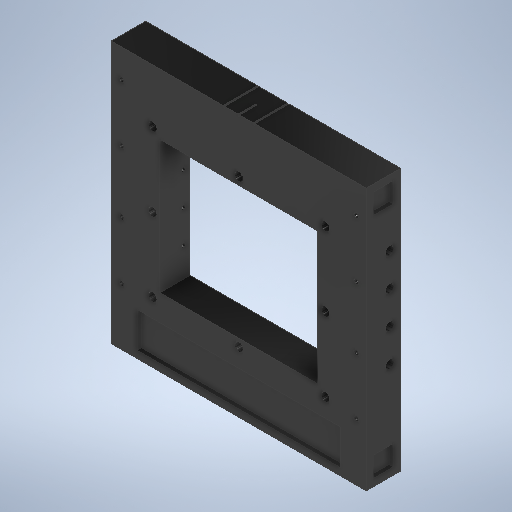
# Autodesk Inventor part: 22024_08_2110_Reaktorkorpus_hinten
Saved by Autodesk Inventor 2025.1 (Build 291241000, 241)
## iProperties
Created: 2020-09-23
Part Number: 22024_08_2110_Reaktorkorpus_hinten
Material: Acetalharz, Weiß
Document SubType Name: Modeling
Designer: Daniel
Density: 1.425 g/cm^3
Appearance: Glatt - Weiß
Author: Daniel
Autodesk Inventor part; units mm, degrees
(part 1 of 3)
ref_plane "YZ Plane" through (0, 0, 0) normal (1, 0, 0) x (0, 1, 0)
ref_plane "XZ Plane" through (0, 0, 0) normal (0, 1, 0) x (-1, 0, 0)
sketch "Skizze1" plane through (0, 0, 0) normal (0, 0, 1) x (1, 0, 0)
  line L0 (89, -91.5) -> (-89, -91.5)
  line L1 (-89, -91.5) -> (-89, 91.5)
  line L2 (-89, 91.5) -> (89, 91.5)
  line L3 (89, 91.5) -> (89, -91.5)
  line L4 (89, -91.5) -> (-89, 91.5) construction
  line L5 (-89, -91.5) -> (89, 91.5) construction
  point P0 (0, 0)
  dimension "d0" = 183
  dimension "d1" = 178
  constraints: 12 end point, 2 midpoint, 2 parallel, 1 horizontal, 1 perpendicular
  measures "d0" distance of L0.end L1.end
  measures "d1" distance of L1.end L2.end
extrude "Extrusion1" add sketch "Skizze1" along normal blind 24
sketch "Skizze2" plane through (0, 0, 24) normal (0, 0, 1) x (1, 0, 0)
  line L0 (-89, 91.5) -> (-89, -91.5) projected
  line L1 (-89, -91.5) -> (89, -91.5) projected
  line L2 (-89, 91.5) -> (89, 91.5)
  line L3 (89, 91.5) -> (89, -91.5)
  line L4 (89, -91.5) -> (-89, -91.5)
  line L5 (-89, -91.5) -> (-89, 91.5)
  line L6 (87, -89.5) -> (-87, -89.5)
  line L7 (-87, -89.5) -> (-87, 89.5)
  line L8 (-87, 89.5) -> (87, 89.5)
  line L9 (87, 89.5) -> (87, -89.5)
  line L10 (87, -89.5) -> (-87, 89.5) construction
  line L11 (-87, -89.5) -> (87, 89.5) construction
  line L12 (-70, -89.5) -> (70, -89.5)
  line L13 (70, -89.5) -> (70, 89.5)
  line L14 (70, 89.5) -> (-70, 89.5)
  line L15 (-70, 89.5) -> (-70, -89.5)
  line L16 (-70, -89.5) -> (70, 89.5) construction
  line L17 (70, -89.5) -> (-70, 89.5) construction
  line L18 (-65, -89.5) -> (65, -89.5)
  line L19 (65, -89.5) -> (65, 89.5)
  line L20 (65, 89.5) -> (-65, 89.5)
  line L21 (-65, 89.5) -> (-65, -89.5)
  line L22 (-65, -89.5) -> (65, 89.5) construction
  line L23 (65, -89.5) -> (-65, 89.5) construction
  line L24 (-65, 89.5) -> (-65, 91.5)
  line L25 (89, 91.5) -> (-89, 91.5) projected
  line L26 (-65, -89.5) -> (-65, -91.5)
  line L27 (65, -89.5) -> (65, -91.5)
  line L28 (65, 89.5) -> (65, 91.5)
  line L29 (89, -91.5) -> (89, 91.5) projected
  line L30 (-89, -91.5) -> (89, -91.5)
  line L31 (89, -91.5) -> (89, -86.5)
  line L32 (89, -86.5) -> (-89, -86.5)
  line L33 (-89, -86.5) -> (-89, -91.5)
  point P0 (0, 0)
  point P1 (70, -89.5)
  point P2 (87, -86.5)
  point P3 (70, -86.5)
  point P4 (-70, -86.5)
  point P5 (-87, -86.5)
  dimension "d4" = 2
  dimension "d5" = 2
  dimension "d6" = 17
  dimension "d7" = 24
  dimension "d10" = 5
  constraints: 60 end point, 11 parallel, 9 point on line, 6 midpoint, 6 perpendicular, 5 horizontal
  measures "d4" distance between parallel lines of L2 L8
  measures "d5" distance between parallel lines of L0 L7
  measures "d6" distance between parallel lines of L9 L13
  measures "d7" distance between parallel lines of L19 L3
  measures "d10" distance between parallel lines of L1 L32
extrude "Extrusion2" add sketch "Skizze2" along normal blind 156.5 contours L2 L24 L8 L7 L32 L0 | L32 L7 L6 L26 L1 L0 | L32 L15 L6 L7 | L2 L3 L32 L9 L8 L28 | L21 L32 L15 L8 | L32 L21 L6 L15 | L8 L13 L32 L19 | L27 L6 L9 L32 L3 L1 | L32 L13 L6 L19 | L9 L6 L13 L32
sketch "Skizze3" plane through (-89, 91.5, 0) normal (0, 1, 0) x (1, 0, 0)
  line L0 (0, 0) -> (0, -180.5) projected
  line L1 (0, -180.5) -> (55, -235.5)
  line L2 (0, -180.5) -> (24, -180.5) projected
  line L3 (24, -180.5) -> (-22.6667, -227.1667)
  line L4 (154, -24) -> (154, -180.5) projected
  line L5 (154, -180.5) -> (202, -228.5)
  line L6 (178, 0) -> (178, -180.5) projected
  line L7 (178, -180.5) -> (113.5, -245)
  line L8 (178, -180.5) -> (154, -180.5) projected
  line L9 (2, -24) -> (2, -180.5) projected
  line L10 (2, -180.5) -> (13, -191.5)
  line L11 (19, -180.5) -> (9.5, -190)
  line L12 (159, -24) -> (159, -180.5) projected
  line L13 (159, -180.5) -> (169, -189.5)
  line L14 (176, -24) -> (176, -180.5) projected
  line L15 (176, -180.5) -> (165, -191.5)
  point P0 (89, 0)
  point P1 (167.9474, -188.5526)
  point P2 (166, -192.5)
  point P3 (10.5, -189)
  point P4 (12, -192.5)
  dimension "d11" = 45
  dimension "d12" = 45
  dimension "d13" = 45
  dimension "d14" = 45
  constraints: 16 end point, 5 point on line, 3 perpendicular
  measures "d11" angle of L3 L2
  measures "d12" angle of L1 L2
  measures "d13" angle of L5 L8
  measures "d14" angle of L8 L7
extrude "Extrusion3" add sketch "Skizze3" against normal up to surface (183 mm away) contours L2 L10 L11 L1 | L11 L10 L3 L1 | L11 L2 L3 L10 | L8 L13 L15 L5 | L15 L13 L7 L5 | L15 L8 L7 L13
sketch "Skizze4" plane through (-89, -91.5, 0) normal (0, -1, 0) x (1, 0, 0)
  line L0 (19, 180.5) -> (10.5, 189) projected
  line L1 (10.5, 189) -> (19, 180.5)
  line L2 (2, 24) -> (2, 180.5) projected
  line L3 (19, 180.5) -> (2, 180.5)
  line L4 (10.5, 189) -> (2, 180.5) projected
  line L5 (2, 180.5) -> (10.5, 189)
  line L6 (167.9474, 188.5526) -> (159, 180.5) projected
  line L7 (176, 180.5) -> (167.9474, 188.5526) projected
  line L8 (159, 180.5) -> (167.9474, 188.5526)
  line L9 (159, 180.5) -> (176, 180.5) projected
  line L10 (167.9474, 188.5526) -> (176, 180.5)
  line L11 (176, 180.5) -> (159, 180.5)
  point P0 (89, 0)
  constraints: 12 end point, 2 collinear, 1 horizontal, 1 perpendicular
extrude "Extrusion4" add sketch "Skizze4" against normal blind 5
sketch "Skizze5" plane through (-89, 91.5, 0) normal (0, 1, 0) x (1, 0, 0)
  line L0 (10.5, -189) -> (2, -180.5) projected
  line L1 (2, -180.5) -> (10.5, -189)
  line L2 (10.5, -189) -> (19, -180.5)
  line L3 (19, -180.5) -> (10.5, -189) projected
  line L4 (2, -180.5) -> (19, -180.5)
  line L5 (167.9474, -188.5526) -> (159, -180.5) projected
  line L6 (176, -180.5) -> (167.9474, -188.5526) projected
  line L7 (159, -180.5) -> (176, -180.5)
  line L8 (159, -180.5) -> (167.9474, -188.5526)
  line L9 (176, -180.5) -> (167.9474, -188.5526)
  point P0 (89, 0)
  constraints: 13 end point, 3 collinear, 2 horizontal
extrude "Extrusion5" add sketch "Skizze5" against normal blind 2
sketch "Skizze6" plane through (0, 0, 0) normal (0, 0, -1) x (-1, 0, 0)
  line L0 (89, 91.5) -> (89, -91.5) projected
  line L1 (-89, -91.5) -> (89, -91.5)
  line L2 (89, -91.5) -> (89, -86.5)
  line L3 (89, -86.5) -> (-89, -86.5)
  line L4 (-89, -86.5) -> (-89, -91.5)
  line L5 (-89, -86.5) -> (89, -86.5)
  line L6 (89, -86.5) -> (89, -62.5)
  line L7 (89, -62.5) -> (-89, -62.5)
  line L8 (-89, -62.5) -> (-89, -86.5)
  line L9 (-89, -91.5) -> (-89, 91.5) projected
  line L10 (-89, 91.5) -> (89, 91.5)
  line L11 (89, 91.5) -> (89, 67.5)
  line L12 (89, 67.5) -> (-89, 67.5)
  line L13 (-89, 67.5) -> (-89, 91.5)
  line L14 (-89, 67.5) -> (89, -62.5) construction
  line L15 (89, 67.5) -> (-89, -62.5) construction
  line L16 (-75.35, -64) -> (75.35, -64)
  line L17 (75.35, -64) -> (75.35, 69)
  line L18 (75.35, 69) -> (-75.35, 69)
  line L19 (-75.35, 69) -> (-75.35, -64)
  line L20 (-75.35, -64) -> (75.35, 69) construction
  line L21 (75.35, -64) -> (-75.35, 69) construction
  point P0 (0, 0)
  point P1 (0, 2.5)
  dimension "d21" = 5
  dimension "d22" = 24
  dimension "d23" = 24
  dimension "d24" = 150.7
  dimension "d25" = 133
  constraints: 40 end point, 8 parallel, 4 horizontal, 4 perpendicular, 3 midpoint, 3 point on line
  measures "d21" distance between parallel lines of L1 L3
  measures "d22" distance between parallel lines of L3 L7
  measures "d23" distance between parallel lines of L12 L10
  measures "d24" distance of L17.end L18.end
  measures "d25" distance of L18.end L16.start
extrude "Extrusion6" cut sketch "Skizze6" against normal blind 3 contours L17 L7 L19 L12 | L12 L19 L18 L17 | L17 L16 L19 L7
sketch "Skizze7" plane through (0, 0, 3) normal (0, 0, -1) x (-1, 0, 0)
  line L0 (-75.35, 69) -> (75.35, -64) construction
  line L1 (75.35, -64) -> (75.35, 69) construction
  line L2 (75.35, 69) -> (-75.35, -64) construction
  line L3 (-55.1, 48.75) -> (55.1, 48.75)
  line L4 (55.1, 48.75) -> (55.1, -43.75)
  line L5 (55.1, -43.75) -> (-55.1, -43.75)
  line L6 (-55.1, -43.75) -> (-55.1, 48.75)
  line L7 (-55.1, 48.75) -> (55.1, -43.75) construction
  line L8 (55.1, 48.75) -> (-55.1, -43.75) construction
  line L9 (-75.35, 69) -> (75.35, 69) projected
  line L10 (75.35, -64) -> (-75.35, -64) projected
  line L11 (0, 2.5) -> (75.35, 2.5) construction
  line L12 (-75.35, -64) -> (-75.35, 69) projected
  line L13 (0, 2.5) -> (-75.35, 2.5) construction
  line L14 (-60.35, -49) -> (-60.35, 55.7618) construction
  line L15 (0, -49) -> (-60.35, -49) construction
  line L16 (0, -49) -> (60.35, -49) construction
  line L17 (60.35, -49) -> (60.35, 2.5) construction
  line L18 (60.35, 2.5) -> (60.35, 54) construction
  line L19 (60.35, 54) -> (0, 54) construction
  line L20 (0, 54) -> (60.35, 54) construction
  circle A0 centre (0, 54) radius 1.7
  circle A1 centre (60.35, 54) radius 1.7
  circle A2 centre (60.35, 2.5) radius 1.7
  circle A3 centre (60.35, -49) radius 1.7
  circle A4 centre (0, -49) radius 1.7
  circle A5 centre (-60.35, -49) radius 1.7
  circle A6 centre (-60.35, 2.5) radius 1.7
  line L21 (0, 54) -> (-60.35, 54) construction
  circle A7 centre (-60.35, 54) radius 1.7
  point P0 (-60.35, 2.5)
  point P1 (60.35, 2.5)
  point P2 (0, 0)
  dimension "d105" = 92.5
  dimension "d106" = 110.2
  dimension "d107" = 15
  dimension "d108" = 15
  dimension "d109" = 15
  dimension "d110" = 15
  dimension "d112" = 3.4
  dimension "d113" = 3.4
  dimension "d114" = 3.4
  dimension "d115" = 3.4
  dimension "d116" = 3.4
  dimension "d117" = 3.4
  dimension "d118" = 3.4
  dimension "d119" = 0
  dimension "d120" = 0
  dimension "d121" = 0
  dimension "d122" = 0
  dimension "d123" = 0
  dimension "d125" = 0
  dimension "d126" = 0
  dimension "d127" = 0
  dimension "d128" = 0
  dimension "d129" = 0
  dimension "d130" = 0
  dimension "d131" = 3.4
  dimension "d132" = 120.7
  dimension "d133" = 103
  dimension "d134" = 2.5
  constraints: 38 end point, 8 centre point, 7 point on line, 5 midpoint, 4 perpendicular, 2 horizontal, 2 parallel, 2 vertical
  measures "d105" distance of L5.end L3.start
  measures "d106" distance of L3.start L3.end
  measures "d107" distance from line of L9 L19.end
  measures "d108" distance from line of L10 L15.start
  measures "d109" distance from line of L17.end L1
  measures "d110" distance from line of L12 point (-60.35, 2.5)
  measures "d112" diameter of A0
  measures "d113" diameter of A1
  measures "d114" diameter of A2
  measures "d115" diameter of A3
  measures "d116" diameter of A4
  measures "d117" diameter of A5
  measures "d118" diameter of A6
  measures "d119" distance of L21.start L19.end
  measures "d120" distance of point (-60.35, 2.5) A6.centre
  measures "d121" distance of A4.centre L15.start
  measures "d122" distance of L17.end A2.centre
  measures "d123" distance from line of A6.centre L14
  measures "d125" distance of A5.centre L14.start
  measures "d126" distance of A5.centre L14.start
  measures "d127" distance of A3.centre L16.end
  measures "d128" distance of L16.end A3.centre
  measures "d129" distance of L18.end A1.centre
  measures "d130" distance of L18.end A1.centre
  measures "d131" diameter of A7
  measures "d132" distance of A2.centre A6.centre
  measures "d133" distance of A4.centre L21.start
  measures "d134" distance of point (0, 0) L11.start
extrude "Extrusion7" cut sketch "Skizze7" against normal through all
sketch "Skizze8" plane through (-89, -91.5, 0) normal (0, -1, 0) x (1, 0, 0)
  line L0 (0, 0) -> (0, 180.5) projected
  line L1 (24, 24) -> (24, 180.5) projected
  line L2 (0, 180.5) -> (24, 180.5)
  line L3 (24, 180.5) -> (24, 156.5)
  line L4 (24, 156.5) -> (0, 156.5)
  line L5 (0, 156.5) -> (0, 180.5)
  line L6 (154, 24) -> (154, 180.5) projected
  line L7 (178, 0) -> (178, 180.5) projected
  line L8 (154, 180.5) -> (178, 180.5)
  line L9 (178, 180.5) -> (178, 156.5)
  line L10 (178, 156.5) -> (154, 156.5)
  line L11 (154, 156.5) -> (154, 180.5)
  line L12 (178, 0) -> (0, 0) projected
  line L13 (178, 0) -> (154, 0)
  line L14 (154, 0) -> (154, 24)
  line L15 (154, 24) -> (178, 24)
  line L16 (178, 24) -> (178, 0)
  line L17 (0, 0) -> (24, 0)
  line L18 (24, 0) -> (24, 24)
  line L19 (24, 24) -> (0, 24)
  line L20 (0, 24) -> (0, 0)
  line L21 (0, 180.5) -> (24, 156.5) construction
  line L22 (24, 180.5) -> (0, 156.5) construction
  line L23 (154, 180.5) -> (178, 156.5) construction
  line L24 (178, 180.5) -> (154, 156.5) construction
  line L25 (154, 24) -> (178, 0) construction
  line L26 (178, 24) -> (154, 0) construction
  line L27 (0, 24) -> (24, 0) construction
  line L28 (24, 24) -> (0, 0) construction
  line L29 (5, 5) -> (19, 5)
  line L30 (19, 5) -> (19, 19)
  line L31 (19, 19) -> (5, 19)
  line L32 (5, 19) -> (5, 5)
  line L33 (5, 5) -> (19, 19) construction
  line L34 (19, 5) -> (5, 19) construction
  line L35 (159, 19) -> (173, 19)
  line L36 (173, 19) -> (173, 5)
  line L37 (173, 5) -> (159, 5)
  line L38 (159, 5) -> (159, 19)
  line L39 (159, 19) -> (173, 5) construction
  line L40 (173, 19) -> (159, 5) construction
  line L41 (159, 175.5) -> (173, 175.5)
  line L42 (173, 175.5) -> (173, 161.5)
  line L43 (173, 161.5) -> (159, 161.5)
  line L44 (159, 161.5) -> (159, 175.5)
  line L45 (159, 175.5) -> (173, 161.5) construction
  line L46 (173, 175.5) -> (159, 161.5) construction
  line L47 (5, 175.5) -> (19, 175.5)
  line L48 (19, 175.5) -> (19, 161.5)
  line L49 (19, 161.5) -> (5, 161.5)
  line L50 (5, 161.5) -> (5, 175.5)
  line L51 (5, 175.5) -> (19, 161.5) construction
  line L52 (19, 175.5) -> (5, 161.5) construction
  point P0 (89, 0)
  point P1 (12, 12)
  point P2 (166, 12)
  point P3 (166, 168.5)
  point P4 (12, 168.5)
  dimension "d38" = 24
  dimension "d39" = 24
  dimension "d40" = 14
  dimension "d41" = 14
  dimension "d187" = 14
  constraints: 96 end point, 16 parallel, 13 midpoint, 11 perpendicular, 10 point on line, 8 horizontal
  measures "d38" distance of L0.end L2.end
  measures "d39" distance between parallel lines of L4 L2
  measures "d40" distance of L47.start L47.end
  measures "d41" distance of L42.end L43.end
  measures "d187" distance of L35.start L35.end
extrude "Extrusion8" cut sketch "Skizze8" against normal blind 3 contours L32 L31 L30 L29 | L35 L36 L37 L38 | L41 L42 L43 L44 | L47 L48 L49 L50
ref_plane "Arbeitsebene1" through (77, 91.5, 192.5) normal (0, 0, -1) x (0, -1, 0)
sketch "Skizze9" plane through (77, 91.5, 192.5) normal (0, 0, -1) x (0, -1, 0)
  line L0 (183, -12) -> (0, -12) projected
  line L1 (183, 166) -> (178, 166)
  line L2 (178, 166) -> (178, -12)
  line L3 (178, -12) -> (183, -12)
  line L4 (183, -12) -> (183, 166)
  line L5 (183, 166) -> (183, -12) construction
  line L6 (183, 166) -> (178, -12) construction
  line L7 (183, -12) -> (178, 166) construction
  line L8 (180.5, 77) -> (134.2573, 77) construction
  line L9 (134.2573, 24.15) -> (134.2573, 129.85) construction
  line L10 (190.25, 79) -> (165.75, 79)
  line L11 (165.75, 79) -> (165.75, 75)
  line L12 (165.75, 75) -> (190.25, 75)
  line L13 (190.25, 75) -> (190.25, 79)
  line L14 (190.25, 79) -> (165.75, 75) construction
  line L15 (165.75, 79) -> (190.25, 75) construction
  line L16 (153.5, 148) -> (178, 148)
  line L17 (178, 148) -> (178, 6)
  line L18 (178, 6) -> (153.5, 6)
  line L19 (153.5, 6) -> (153.5, 148)
  line L20 (153.5, 148) -> (178, 6) construction
  line L21 (178, 148) -> (153.5, 6) construction
  line L22 (183, 142) -> (0, 142) projected
  line L23 (0, 12) -> (183, 12) projected
  point P0 (91.5, 77)
  point P1 (178, 77)
  point P2 (165.75, 77)
  point P3 (178, 148)
  dimension "d44" = 5
  dimension "d45" = 24.5
  dimension "d46" = 6
  dimension "d47" = 6
  constraints: 38 end point, 8 midpoint, 6 parallel, 3 horizontal, 3 perpendicular, 3 point on line
  measures "d44" distance between parallel lines of L4 L2
  measures "d45" distance of L11.end L12.end
  measures "d46" distance between parallel lines of L16 L22
  measures "d47" distance between parallel lines of L23 L18
extrude "Extrusion9" cut sketch "Skizze9" along normal up to surface (168.5 mm away) contours L18 L19 L23 L2 | L23 L19 L22 L2 L10 L11 L12 | L12 L11 L10 L2 | L19 L16 L2 L22
sketch "Skizze10" plane through (0, 0, 24) normal (0, 0, 1) x (1, 0, 0)
  line L0 (-71, -86.5) -> (-71, -62) construction
  line L1 (78.9474, -86.5) -> (71, -86.5) construction
  line L2 (-71, -62) -> (71, -86.5) construction
  line L3 (70, -62) -> (70, 89.5) construction
  line L4 (71, -86.5) -> (71, -61.9796) construction
  line L5 (71, -61.9796) -> (-71, -86.5) construction
  line L6 (-87, -86.5) -> (-65, -86.5) projected
  line L7 (-73.9133, -86.5) -> (-73.9133, -62)
  line L8 (-77, 91.5) -> (-77, -91.5) projected
  line L9 (-71, -62) -> (-65, -62) projected
  line L10 (-71, -62) -> (71, -62)
  line L11 (71, -62) -> (71, -86.5)
  line L12 (71, -86.5) -> (-71, -86.5)
  line L13 (-71, -86.5) -> (-71, -62)
  point P0 (0, 0)
  point P1 (0, -74.2398)
  constraints: 16 end point, 4 parallel, 1 horizontal, 1 midpoint, 1 perpendicular, 1 point on line
extrude "Extrusion10" cut sketch "Skizze10" against normal blind 3
sketch "Skizze11" plane through (-89, 91.5, 0) normal (0, 1, 0) x (1, 0, 0)
  line L0 (0, -180.5) -> (12, -192.5) projected
  line L1 (178, 0) -> (178, -180.5) projected
  line L2 (0, -180.5) -> (178, -180.5)
  line L3 (178, -180.5) -> (178, -178.5)
  line L4 (178, -178.5) -> (0, -178.5)
  line L5 (0, -178.5) -> (0, -180.5)
  line L6 (0, -180.5) -> (178, -178.5) construction
  line L7 (178, -180.5) -> (0, -178.5) construction
  line L8 (89, -179.5) -> (89, -173) construction
  line L9 (79, -190.75) -> (99, -190.75) construction
  line L10 (99, -190.75) -> (99, -166.25) construction
  line L11 (99, -166.25) -> (79, -166.25) construction
  line L12 (79, -166.25) -> (79, -190.75) construction
  line L13 (79, -190.75) -> (99, -166.25) construction
  line L14 (99, -190.75) -> (79, -166.25) construction
  line L15 (21, -154) -> (157, -154)
  line L16 (157, -154) -> (157, -178.5)
  line L17 (157, -178.5) -> (21, -178.5)
  line L18 (21, -178.5) -> (21, -154)
  line L19 (21, -154) -> (157, -178.5) construction
  line L20 (157, -154) -> (21, -178.5) construction
  line L21 (154, -24) -> (154, -180.5) projected
  line L22 (24, -24) -> (24, -180.5) projected
  point P0 (89, 0)
  point P1 (89, -178.5)
  point P2 (89, -166.25)
  point P3 (21, -178.5)
  dimension "d52" = 2
  dimension "d53" = 24.5
  dimension "d54" = 3
  dimension "d55" = 3
  constraints: 38 end point, 7 midpoint, 6 parallel, 3 horizontal, 3 perpendicular, 3 point on line, 1 vertical
  measures "d52" distance between parallel lines of L2 L4
  measures "d53" distance of L9.end L10.end
  measures "d54" distance between parallel lines of L16 L21
  measures "d55" distance between parallel lines of L18 L22
extrude "Extrusion11" cut sketch "Skizze11" against normal blind 181 contours L4 L21 L15 L16 | L4 L22 L15 L21 | L4 L18 L15 L22
sketch "Skizze12" plane through (77, 91.5, 192.5) normal (0, 0, -1) x (0, -1, 0)
  line L0 (178, 148) -> (153.5, 148) construction
  line L1 (153.5, 6) -> (178, 6) construction
  line L2 (153.5, 148) -> (178, 6) construction
  line L3 (178, 6) -> (153.5, 6) construction
  line L4 (153.5, 6) -> (178, 148) construction
  line L5 (165.75, 77) -> (145.75, 77) construction
  line L6 (145.75, 77) -> (145.75, 9) construction
  line L7 (0, 9) -> (153.5, 9) construction
  line L8 (145.75, 9) -> (145.75, 145) construction
  line L9 (0, 145) -> (153.5, 145) construction
  line L10 (135.75, 145) -> (135.75, 9) construction
  line L11 (135.75, 9) -> (125.75, 9) construction
  line L12 (125.75, 9) -> (125.75, 145) construction
  line L13 (115.75, 145) -> (115.75, 9) construction
  line L14 (115.75, 9) -> (105.75, 9) construction
  line L15 (105.75, 9) -> (105.75, 145) construction
  line L16 (95.75, 145) -> (95.75, 9) construction
  line L17 (95.75, 9) -> (85.75, 9) construction
  line L18 (85.75, 9) -> (85.75, 145) construction
  line L19 (75.75, 145) -> (75.75, 9) construction
  line L20 (75.75, 9) -> (65.75, 9) construction
  line L21 (65.75, 9) -> (65.75, 145) construction
  line L22 (55.75, 145) -> (55.75, 9) construction
  line L23 (45.75, 145) -> (45.75, 9) construction
  line L24 (35.75, 9) -> (35.75, 145) construction
  line L25 (25.75, 145) -> (25.75, 9) construction
  line L26 (15.75, 9) -> (15.75, 145) construction
  line L27 (149.75, 139) -> (141.75, 139)
  line L28 (141.75, 139) -> (141.75, 145)
  line L29 (141.75, 145) -> (149.75, 145)
  line L30 (149.75, 145) -> (149.75, 139)
  line L31 (149.75, 139) -> (141.75, 145) construction
  line L32 (141.75, 139) -> (149.75, 145) construction
  line L33 (141.75, 145) -> (143.75, 142)
  line L34 (149.75, 145) -> (147.75, 142)
  line L35 (153.5, 142) -> (0, 142) projected
  line L36 (143.75, 142) -> (147.75, 142)
  line L37 (0, 12) -> (153.5, 12) projected
  line L38 (149.75, 15) -> (141.75, 15)
  line L39 (141.75, 15) -> (141.75, 9)
  line L40 (141.75, 9) -> (149.75, 9)
  line L41 (149.75, 9) -> (149.75, 15)
  line L42 (149.75, 15) -> (141.75, 9) construction
  line L43 (141.75, 15) -> (149.75, 9) construction
  line L44 (149.75, 9) -> (147.75, 12)
  line L45 (141.75, 9) -> (143.75, 12)
  line L46 (143.75, 12) -> (147.75, 12)
  line L47 (131.75, 145) -> (139.75, 145)
  line L48 (131.75, 145) -> (133.75, 142)
  line L49 (139.75, 145) -> (137.75, 142)
  line L50 (133.75, 142) -> (137.75, 142)
  line L51 (131.75, 9) -> (139.75, 9)
  line L52 (139.75, 9) -> (137.75, 12)
  line L53 (131.75, 9) -> (133.75, 12)
  line L54 (133.75, 12) -> (137.75, 12)
  line L55 (121.75, 145) -> (129.75, 145)
  line L56 (121.75, 145) -> (123.75, 142)
  line L57 (129.75, 145) -> (127.75, 142)
  line L58 (123.75, 142) -> (127.75, 142)
  line L59 (121.75, 9) -> (129.75, 9)
  line L60 (129.75, 9) -> (127.75, 12)
  line L61 (121.75, 9) -> (123.75, 12)
  line L62 (123.75, 12) -> (127.75, 12)
  line L63 (111.75, 145) -> (119.75, 145)
  line L64 (111.75, 145) -> (113.75, 142)
  line L65 (119.75, 145) -> (117.75, 142)
  line L66 (113.75, 142) -> (117.75, 142)
  line L67 (111.75, 9) -> (119.75, 9)
  line L68 (119.75, 9) -> (117.75, 12)
  line L69 (111.75, 9) -> (113.75, 12)
  line L70 (113.75, 12) -> (117.75, 12)
  line L71 (101.75, 145) -> (109.75, 145)
  line L72 (101.75, 145) -> (103.75, 142)
  line L73 (109.75, 145) -> (107.75, 142)
  line L74 (103.75, 142) -> (107.75, 142)
  line L75 (101.75, 9) -> (109.75, 9)
  line L76 (109.75, 9) -> (107.75, 12)
  line L77 (101.75, 9) -> (103.75, 12)
  line L78 (103.75, 12) -> (107.75, 12)
  line L79 (91.75, 145) -> (99.75, 145)
  line L80 (91.75, 145) -> (93.75, 142)
  line L81 (99.75, 145) -> (97.75, 142)
  line L82 (93.75, 142) -> (97.75, 142)
  line L83 (91.75, 9) -> (99.75, 9)
  line L84 (99.75, 9) -> (97.75, 12)
  line L85 (91.75, 9) -> (93.75, 12)
  line L86 (93.75, 12) -> (97.75, 12)
  line L87 (81.75, 145) -> (89.75, 145)
  line L88 (81.75, 145) -> (83.75, 142)
  line L89 (89.75, 145) -> (87.75, 142)
  line L90 (83.75, 142) -> (87.75, 142)
  line L91 (81.75, 9) -> (89.75, 9)
  line L92 (89.75, 9) -> (87.75, 12)
  line L93 (81.75, 9) -> (83.75, 12)
  line L94 (83.75, 12) -> (87.75, 12)
  line L95 (71.75, 145) -> (79.75, 145)
  line L96 (71.75, 145) -> (73.75, 142)
  line L97 (79.75, 145) -> (77.75, 142)
  line L98 (73.75, 142) -> (77.75, 142)
  line L99 (71.75, 9) -> (79.75, 9)
  line L100 (79.75, 9) -> (77.75, 12)
  line L101 (71.75, 9) -> (73.75, 12)
  line L102 (73.75, 12) -> (77.75, 12)
  line L103 (61.75, 145) -> (69.75, 145)
  line L104 (61.75, 145) -> (63.75, 142)
  line L105 (69.75, 145) -> (67.75, 142)
  line L106 (63.75, 142) -> (67.75, 142)
  line L107 (61.75, 9) -> (69.75, 9)
  line L108 (69.75, 9) -> (67.75, 12)
  line L109 (61.75, 9) -> (63.75, 12)
  line L110 (63.75, 12) -> (67.75, 12)
  line L111 (51.75, 145) -> (59.75, 145)
  line L112 (51.75, 145) -> (53.75, 142)
  line L113 (59.75, 145) -> (57.75, 142)
  line L114 (53.75, 142) -> (57.75, 142)
  line L115 (51.75, 9) -> (59.75, 9)
  line L116 (59.75, 9) -> (57.75, 12)
  line L117 (51.75, 9) -> (53.75, 12)
  line L118 (53.75, 12) -> (57.75, 12)
  line L119 (41.75, 145) -> (49.75, 145)
  line L120 (41.75, 145) -> (43.75, 142)
  line L121 (49.75, 145) -> (47.75, 142)
  line L122 (43.75, 142) -> (47.75, 142)
  line L123 (41.75, 9) -> (49.75, 9)
  line L124 (49.75, 9) -> (47.75, 12)
  line L125 (41.75, 9) -> (43.75, 12)
  line L126 (43.75, 12) -> (47.75, 12)
  line L127 (31.75, 145) -> (39.75, 145)
  line L128 (31.75, 145) -> (33.75, 142)
  line L129 (39.75, 145) -> (37.75, 142)
  line L130 (33.75, 142) -> (37.75, 142)
  line L131 (31.75, 9) -> (39.75, 9)
  line L132 (39.75, 9) -> (37.75, 12)
  line L133 (31.75, 9) -> (33.75, 12)
  line L134 (33.75, 12) -> (37.75, 12)
  line L135 (21.75, 145) -> (29.75, 145)
  line L136 (21.75, 145) -> (23.75, 142)
  line L137 (29.75, 145) -> (27.75, 142)
  line L138 (23.75, 142) -> (27.75, 142)
  line L139 (21.75, 9) -> (29.75, 9)
  line L140 (29.75, 9) -> (27.75, 12)
  line L141 (21.75, 9) -> (23.75, 12)
  line L142 (23.75, 12) -> (27.75, 12)
  line L143 (11.75, 145) -> (19.75, 145)
  line L144 (11.75, 145) -> (13.75, 142)
  line L145 (19.75, 145) -> (17.75, 142)
  line L146 (13.75, 142) -> (17.75, 142)
  line L147 (11.75, 9) -> (19.75, 9)
  line L148 (19.75, 9) -> (17.75, 12)
  line L149 (11.75, 9) -> (13.75, 12)
  line L150 (13.75, 12) -> (17.75, 12)
  point P0 (91.5, 77)
  point P1 (145.75, 142)
  point P2 (145.75, 12)
  point P3 (135.75, 12)
  point P4 (125.75, 12)
  point P5 (115.75, 12)
  point P6 (105.75, 12)
  point P7 (95.75, 12)
  point P8 (85.75, 12)
  point P9 (75.75, 12)
  point P10 (65.75, 12)
  point P11 (55.75, 12)
  point P12 (45.75, 12)
  point P13 (35.75, 12)
  point P14 (25.75, 12)
  point P15 (15.75, 12)
  point P16 (135.75, 142)
  point P17 (125.75, 142)
  point P18 (115.75, 142)
  point P19 (105.75, 142)
  point P20 (95.75, 142)
  point P21 (85.75, 142)
  point P22 (75.75, 142)
  point P23 (65.75, 142)
  point P24 (55.75, 142)
  point P25 (45.75, 142)
  point P26 (35.75, 142)
  point P27 (25.75, 142)
  point P28 (15.75, 142)
  point P29 (125.75, 145)
  point P30 (115.75, 145)
  point P31 (105.75, 145)
  point P32 (95.75, 145)
  point P33 (85.75, 145)
  point P34 (75.75, 145)
  point P35 (65.75, 145)
  point P36 (35.75, 145)
  point P37 (25.75, 145)
  point P38 (15.75, 145)
  point P39 (13.75, 142)
  point P40 (17.75, 142)
  point P41 (23.75, 142)
  point P42 (27.75, 142)
  point P43 (33.75, 142)
  point P44 (37.75, 142)
  point P45 (17.75, 12)
  point P46 (13.75, 12)
  point P47 (27.75, 12)
  point P48 (23.75, 12)
  point P49 (37.75, 12)
  point P50 (33.75, 12)
  point P51 (43.75, 142)
  point P52 (47.75, 142)
  point P53 (53.75, 142)
  point P54 (57.75, 142)
  point P55 (63.75, 142)
  point P56 (67.75, 142)
  point P57 (73.75, 142)
  point P58 (77.75, 142)
  point P59 (83.75, 142)
  point P60 (107.75, 142)
  point P61 (43.75, 12)
  point P62 (57.75, 12)
  point P63 (53.75, 12)
  point P64 (63.75, 12)
  point P65 (87.75, 12)
  point P66 (97.75, 12)
  point P67 (93.75, 12)
  point P68 (107.75, 12)
  point P69 (103.75, 12)
  point P70 (113.75, 12)
  point P71 (127.75, 12)
  point P72 (123.75, 12)
  point P73 (117.75, 142)
  point P74 (123.75, 142)
  point P75 (127.75, 142)
  point P76 (133.75, 142)
  point P77 (137.75, 12)
  dimension "d58" = 20
  dimension "d59" = 10
  dimension "d60" = 10
  dimension "d61" = 10
  dimension "d62" = 10
  dimension "d63" = 10
  dimension "d64" = 10
  dimension "d65" = 10
  dimension "d66" = 10
  dimension "d67" = 10
  dimension "d68" = 10
  dimension "d69" = 10
  dimension "d70" = 10
  dimension "d71" = 10
  dimension "d72" = 8
  dimension "d73" = 2
  dimension "d74" = 2
  dimension "d75" = 8
  dimension "d76" = 2
  dimension "d77" = 2
  constraints: 290 end point, 36 point on line, 7 perpendicular, 5 midpoint, 5 parallel, 5 vertical, 4 horizontal, 1 collinear, 32 other
  measures "d58" distance of L5.start L5.end
  measures "d59" distance between parallel lines of L10 L8
  measures "d60" distance between parallel lines of L12 L10
  measures "d61" distance between parallel lines of L13 L12
  measures "d62" distance between parallel lines of L13 L15
  measures "d63" distance between parallel lines of L15 L16
  measures "d64" distance between parallel lines of L18 L16
  measures "d65" distance between parallel lines of L18 L19
  measures "d66" distance between parallel lines of L19 L21
  measures "d67" distance between parallel lines of L21 L22
  measures "d68" distance between parallel lines of L23 L22
  measures "d69" distance between parallel lines of L24 L23
  measures "d70" distance between parallel lines of L25 L24
  measures "d71" distance between parallel lines of L26 L25
  measures "d72" distance of L27.start L27.end
  measures "d73" distance from line of L28 L33.end
  measures "d74" distance from line of L30 L34.end
  measures "d75" distance of L38.start L38.end
  measures "d76" distance from line of L39 L45.end
  measures "d77" distance from line of L41 L44.end
extrude "Extrusion12" cut sketch "Skizze12" along normal blind 114 contours L35 L144 L143 L145 | L35 L136 L135 L137 | L35 L128 L127 L129 | L35 L120 L119 L121 | L35 L112 L111 L113 | L35 L104 L103 L105 | L35 L96 L95 L97 | L35 L88 L87 L89 | L35 L80 L79 L81 | L35 L72 L71 L73 | L35 L64 L63 L65 | L35 L56 L55 L57 | L35 L48 L47 L49 | L34 L35 L33 L29 | L37 L52 L51 L53 | L37 L60 L59 L61 | L37 L68 L67 L69 | L37 L76 L75 L77 | L37 L84 L83 L85 | L37 L92 L91 L93 | L37 L100 L99 L101 | L37 L108 L107 L109 | L37 L116 L115 L117 | L37 L124 L123 L125 | L37 L132 L131 L133 | L37 L140 L139 L141 | L37 L148 L147 L149 | L37 L44 L40 L45
sketch "Skizze13" plane through (-89, 91.5, 0) normal (0, 1, 0) x (1, 0, 0)
  line L0 (0, 0) -> (0, -180.5) projected
  line L1 (178, 0) -> (178, -180.5) projected
  line L2 (0, 0) -> (178, 0)
  line L3 (178, 0) -> (178, -178)
  line L4 (178, -178) -> (0, -178)
  line L5 (0, -178) -> (0, 0)
  line L6 (166, -192.5) -> (178, -180.5) projected
  line L7 (178, -178) -> (166, -178)
  line L8 (166, -178) -> (166, -192.5)
  line L9 (166, -192.5) -> (178, -192.5)
  line L10 (178, -192.5) -> (178, -178)
  line L11 (178, 0) -> (178, -180.5) construction
  line L12 (0, -178) -> (178, 0) construction
  line L13 (178, 0) -> (0, 0) construction
  line L14 (178, 0) -> (0, 0) construction
  line L15 (0, 0) -> (178, -178) construction
  line L16 (166, -89.5) -> (12, -89.5)
  line L17 (12, -89.5) -> (12, -88.5)
  line L18 (12, -88.5) -> (166, -88.5)
  line L19 (166, -88.5) -> (166, -89.5)
  line L20 (166, -89.5) -> (12, -88.5) construction
  line L21 (12, -89.5) -> (166, -88.5) construction
  line L22 (88.5, -166) -> (89.5, -166)
  line L23 (89.5, -166) -> (89.5, -12)
  line L24 (89.5, -12) -> (88.5, -12)
  line L25 (88.5, -12) -> (88.5, -166)
  line L26 (88.5, -166) -> (89.5, -12) construction
  line L27 (89.5, -166) -> (88.5, -12) construction
  line L28 (24, -154) -> (24, -24) projected
  line L29 (154, -154) -> (24, -154)
  line L30 (24, -154) -> (24, -24)
  line L31 (24, -24) -> (154, -24)
  line L32 (154, -24) -> (154, -154)
  line L33 (154, -154) -> (24, -24) construction
  line L34 (24, -154) -> (154, -24) construction
  point P0 (89, 0)
  point P1 (89, -89)
  point P2 (88.5, -88.5)
  point P3 (88.5, -89.5)
  point P4 (89.5, -89.5)
  point P5 (89.5, -88.5)
  dimension "d80" = 178
  dimension "d81" = 14.5
  dimension "d82" = 1
  dimension "d83" = 1
  dimension "d84" = 154
  dimension "d85" = 154
  dimension "d90" = 130
  dimension "d91" = 130
  constraints: 58 end point, 11 equal length, 7 midpoint, 5 horizontal, 5 perpendicular, 1 point on line
  measures "d80" distance between parallel lines of L4 L2
  measures "d81" distance between parallel lines of L4 L9
  measures "d82" distance of L16.end L17.end
  measures "d83" distance of L23.end L24.end
  measures "d84" distance of L24.end L22.start
  measures "d85" distance of L17.end L18.end
  measures "d90" distance of L28.end L31.end
  measures "d91" distance of L29.end L28.end
extrude "Extrusion13" cut sketch "Skizze13" against normal blind 1 contours L16 L32 L18 L19 | L16 L23 L18 L32 | L23 L29 L25 L16 | L16 L25 L18 L23 | L16 L28 L18 L25 | L23 L22 L25 L29 | L18 L25 L31 L23 | L16 L17 L18 L28 | L31 L25 L24 L23
sketch "Skizze14" plane through (-77, -91.5, 192.5) normal (0.7071, 0, 0.7071) x (0.7071, 0, -0.7071)
  line L0 (0.4493, 19.9089) -> (5.7022, 19.9089) construction
  line L1 (5.7022, 19.9089) -> (5.7022, 29.9599) construction
  line L2 (5.7022, 29.9599) -> (0.4493, 29.9599) construction
  line L3 (0.4493, 29.9599) -> (0.4493, 19.9089) construction
  line L4 (0.4923, 49.8867) -> (5.7451, 49.8867) construction
  line L5 (5.7451, 49.8867) -> (5.7451, 46.2392) construction
  line L6 (5.7451, 46.2392) -> (0.4923, 46.2392) construction
  line L7 (0.4923, 46.2392) -> (0.4923, 49.8867) construction
  line L8 (0.1277, 60.4817) -> (5.3805, 60.4817) construction
  line L9 (5.3805, 60.4817) -> (5.3805, 56.8342) construction
  line L10 (5.3805, 56.8342) -> (0.1277, 56.8342) construction
  line L11 (0.1277, 56.8342) -> (0.1277, 60.4817) construction
  line L12 (0.177, 70.1367) -> (5.4298, 70.1367) construction
  line L13 (5.4298, 70.1367) -> (5.4298, 66.4892) construction
  line L14 (5.4298, 66.4892) -> (0.177, 66.4892) construction
  line L15 (0.177, 66.4892) -> (0.177, 70.1367) construction
  line L16 (0.177, 80.1367) -> (5.4298, 80.1367) construction
  line L17 (5.4298, 80.1367) -> (5.4298, 76.4892) construction
  line L18 (5.4298, 76.4892) -> (0.177, 76.4892) construction
  line L19 (0.177, 76.4892) -> (0.177, 80.1367) construction
  line L20 (0.177, 90.1367) -> (5.4298, 90.1367) construction
  line L21 (5.4298, 90.1367) -> (5.4298, 86.4892) construction
  line L22 (5.4298, 86.4892) -> (0.177, 86.4892) construction
  line L23 (0.177, 86.4892) -> (0.177, 90.1367) construction
  line L24 (0.177, 100.1367) -> (5.4298, 100.1367) construction
  line L25 (5.4298, 100.1367) -> (5.4298, 96.4892) construction
  line L26 (5.4298, 96.4892) -> (0.177, 96.4892) construction
  line L27 (0.177, 96.4892) -> (0.177, 100.1367) construction
  line L28 (0.177, 110.1367) -> (5.4298, 110.1367) construction
  line L29 (5.4298, 110.1367) -> (5.4298, 106.4892) construction
  line L30 (5.4298, 106.4892) -> (0.177, 106.4892) construction
  line L31 (0.177, 106.4892) -> (0.177, 110.1367) construction
  line L32 (-0.2126, 120.6134) -> (5.0402, 120.6134) construction
  line L33 (5.0402, 120.6134) -> (5.0402, 116.9659) construction
  line L34 (5.0402, 116.9659) -> (-0.2126, 116.9659) construction
  line L35 (-0.2126, 116.9659) -> (-0.2126, 120.6134) construction
  line L36 (-0.2161, 130.1063) -> (5.0368, 130.1063) construction
  line L37 (5.0368, 130.1063) -> (5.0368, 126.4588) construction
  line L38 (5.0368, 126.4588) -> (-0.2161, 126.4588) construction
  line L39 (-0.2161, 126.4588) -> (-0.2161, 130.1063) construction
  line L40 (-0.2978, 140.1) -> (4.9551, 140.1) construction
  line L41 (4.9551, 140.1) -> (4.9551, 136.4525) construction
  line L42 (4.9551, 136.4525) -> (-0.2978, 136.4525) construction
  line L43 (-0.2978, 136.4525) -> (-0.2978, 140.1) construction
  line L44 (-0.3019, 150.1519) -> (4.9509, 150.1519) construction
  line L45 (4.9509, 150.1519) -> (4.9509, 146.5044) construction
  line L46 (4.9509, 146.5044) -> (-0.3019, 146.5044) construction
  line L47 (-0.3019, 146.5044) -> (-0.3019, 150.1519) construction
  line L48 (-0.2744, 160.1018) -> (4.9784, 160.1018) construction
  line L49 (4.9784, 160.1018) -> (4.9784, 156.4543) construction
  line L50 (4.9784, 156.4543) -> (-0.2744, 156.4543) construction
  line L51 (-0.2744, 156.4543) -> (-0.2744, 160.1018) construction
  line L52 (-0.539, 170.1317) -> (4.1973, 170.1317) construction
  line L53 (4.1973, 170.1317) -> (4.1973, 166.4842) construction
  line L54 (4.1973, 166.4842) -> (-0.539, 166.4842) construction
  line L55 (-0.539, 166.4842) -> (-0.539, 170.1317) construction
  line L56 (0.5265, 39.54) -> (5.7793, 39.54) construction
  line L57 (5.7793, 39.54) -> (5.7793, 35.8925) construction
  line L58 (5.7793, 35.8925) -> (0.5265, 35.8925) construction
  line L59 (0.5265, 35.8925) -> (0.5265, 39.54) construction
  line L60 (8.4853, 5) -> (8.4853, 29.5) projected
  line L61 (12.1672, 16.75) -> (4.8034, 16.75)
  line L62 (4.8034, 16.75) -> (4.8034, 17.75)
  line L63 (4.8034, 17.75) -> (12.1672, 17.75)
  line L64 (12.1672, 17.75) -> (12.1672, 16.75)
  line L65 (12.1672, 16.75) -> (4.8034, 17.75) construction
  line L66 (4.8034, 16.75) -> (12.1672, 17.75) construction
  line L67 (7.3114, 17.75) -> (7.3114, 16.75)
  line L68 (2.9776, 164.5202) -> (0.2945, 164.5202)
  line L69 (0.2945, 164.5202) -> (0.2945, 165.0818)
  line L70 (0.2945, 165.0818) -> (1.2928, 165.0818)
  line L71 (1.2928, 165.0818) -> (1.2928, 168.7678)
  line L72 (1.2928, 168.7678) -> (0.2945, 168.7678)
  line L73 (0.2945, 168.7678) -> (0.2945, 169.2715)
  spline S0 degree 2 poles (0.2945, 169.2715) (0.8605, 169.2715) (1.3954, 169.5924) (1.431, 170.0381) knots 0 0 0 1 2 2 2
  line L74 (1.431, 170.0381) -> (2.0015, 170.0381)
  line L75 (2.0015, 170.0381) -> (2.0015, 165.0818)
  line L76 (2.0015, 165.0818) -> (2.9776, 165.0818)
  line L77 (2.9776, 165.0818) -> (2.9776, 164.5202)
  spline S1 degree 2 poles (7.4659, 166.3031) (7.4659, 165.8796) (7.1851, 165.1621) (6.9488, 164.9214) knots 0 0 0 1 2 2 2
  spline S2 degree 2 poles (6.9488, 164.9214) (6.7037, 164.6673) (6.0886, 164.4044) (5.7187, 164.4044) knots 0 0 0 1 2 2 2
  spline S3 degree 2 poles (5.7187, 164.4044) (5.3488, 164.4044) (4.7381, 164.6539) (4.5064, 164.9035) knots 0 0 0 1 2 2 2
  spline S4 degree 2 poles (4.5064, 164.9035) (4.2211, 165.2022) (3.9002, 166.205) (3.9002, 166.936) knots 0 0 0 1 2 2 2
  spline S5 degree 2 poles (3.9002, 166.936) (3.9002, 167.6535) (4.1944, 168.8079) (4.5019, 169.2358) knots 0 0 0 1 2 2 2
  spline S6 degree 2 poles (4.5019, 169.2358) (4.8005, 169.6548) (5.7454, 170.1227) (6.365, 170.1227) knots 0 0 0 1 2 2 2
  spline S7 degree 2 poles (6.365, 170.1227) (6.5477, 170.1227) (6.8686, 170.0871) (6.989, 170.047) knots 0 0 0 1 2 2 2
  line L78 (6.989, 170.047) -> (6.989, 169.3383)
  line L79 (6.989, 169.3383) -> (6.9578, 169.3383)
  spline S8 degree 2 poles (6.9578, 169.3383) (6.8552, 169.3918) (6.4808, 169.4854) (6.2669, 169.4854) knots 0 0 0 1 2 2 2
  spline S9 degree 2 poles (6.2669, 169.4854) (5.5805, 169.4854) (4.7381, 168.5583) (4.6579, 167.6491) knots 0 0 0 1 2 2 2
  spline S10 degree 2 poles (4.6579, 167.6491) (4.9209, 167.8318) (5.4736, 168.0324) (5.8034, 168.0324) knots 0 0 0 1 2 2 2
  spline S11 degree 2 poles (5.8034, 168.0324) (6.1243, 168.0324) (6.6056, 167.9031) (6.8686, 167.707) knots 0 0 0 1 2 2 2
  spline S12 degree 2 poles (6.8686, 167.707) (7.1717, 167.4797) (7.4659, 166.7755) (7.4659, 166.3031) knots 0 0 0 1 2 2 2
  spline S13 degree 2 poles (6.7171, 166.2719) (6.7171, 166.6106) (6.5388, 167.0697) (6.3427, 167.2301) knots 0 0 0 1 2 2 2
  spline S14 degree 2 poles (6.3427, 167.2301) (6.1956, 167.346) (5.8301, 167.4218) (5.6385, 167.4218) knots 0 0 0 1 2 2 2
  spline S15 degree 2 poles (5.6385, 167.4218) (5.38, 167.4218) (4.8941, 167.2658) (4.6579, 167.1187) knots 0 0 0 1 2 2 2
  spline S16 degree 2 poles (4.6579, 167.1187) (4.6535, 167.0385) (4.6445, 166.8869) (4.6445, 166.771) knots 0 0 0 1 2 2 2
  spline S17 degree 2 poles (4.6445, 166.771) (4.6445, 166.2005) (4.8674, 165.5008) (5.0368, 165.318) knots 0 0 0 1 2 2 2
  spline S18 degree 2 poles (5.0368, 165.318) (5.1928, 165.1442) (5.5315, 165.0061) (5.7231, 165.0061) knots 0 0 0 1 2 2 2
  spline S19 degree 2 poles (5.7231, 165.0061) (6.1689, 165.0061) (6.7171, 165.639) (6.7171, 166.2719) knots 0 0 0 1 2 2 2
  spline S20 degree 2 poles (11.5396, 167.2702) (11.5396, 165.7905) (10.6794, 164.4044) (9.7835, 164.4044) knots 0 0 0 1 2 2 2
  spline S21 degree 2 poles (9.7835, 164.4044) (8.8743, 164.4044) (8.023, 165.8172) (8.023, 167.2658) knots 0 0 0 1 2 2 2
  spline S22 degree 2 poles (8.023, 167.2658) (8.023, 168.7544) (8.8832, 170.1317) (9.7835, 170.1317) knots 0 0 0 1 2 2 2
  spline S23 degree 2 poles (9.7835, 170.1317) (10.6883, 170.1317) (11.5396, 168.7054) (11.5396, 167.2702) knots 0 0 0 1 2 2 2
  spline S24 degree 2 poles (10.5947, 165.5944) (10.7017, 165.8663) (10.7908, 166.7042) (10.7908, 167.2702) knots 0 0 0 1 2 2 2
  spline S25 degree 2 poles (10.7908, 167.2702) (10.7908, 167.8363) (10.7017, 168.6697) (10.5902, 168.9505) knots 0 0 0 1 2 2 2
  spline S26 degree 2 poles (10.5902, 168.9505) (10.4788, 169.2313) (10.0911, 169.521) (9.7835, 169.521) knots 0 0 0 1 2 2 2
  spline S27 degree 2 poles (9.7835, 169.521) (9.476, 169.521) (9.0793, 169.2313) (8.9634, 168.9416) knots 0 0 0 1 2 2 2
  spline S28 degree 2 poles (8.9634, 168.9416) (8.852, 168.6608) (8.7718, 167.8051) (8.7718, 167.2658) knots 0 0 0 1 2 2 2
  spline S29 degree 2 poles (8.7718, 167.2658) (8.7718, 166.6864) (8.8431, 165.9108) (8.959, 165.6078) knots 0 0 0 1 2 2 2
  spline S30 degree 2 poles (8.959, 165.6078) (9.0659, 165.3225) (9.4626, 165.015) (9.7835, 165.015) knots 0 0 0 1 2 2 2
  spline S31 degree 2 poles (9.7835, 165.015) (10.0866, 165.015) (10.4833, 165.3047) (10.5947, 165.5944) knots 0 0 0 1 2 2 2
  line L80 (3.2422, 154.4903) -> (0.559, 154.4903)
  line L81 (0.559, 154.4903) -> (0.559, 155.0519)
  line L82 (0.559, 155.0519) -> (1.5574, 155.0519)
  line L83 (1.5574, 155.0519) -> (1.5574, 158.7379)
  line L84 (1.5574, 158.7379) -> (0.559, 158.7379)
  line L85 (0.559, 158.7379) -> (0.559, 159.2416)
  spline S32 degree 2 poles (0.559, 159.2416) (1.1251, 159.2416) (1.6599, 159.5625) (1.6956, 160.0082) knots 0 0 0 1 2 2 2
  line L86 (1.6956, 160.0082) -> (2.2661, 160.0082)
  line L87 (2.2661, 160.0082) -> (2.2661, 155.0519)
  line L88 (2.2661, 155.0519) -> (3.2422, 155.0519)
  line L89 (3.2422, 155.0519) -> (3.2422, 154.4903)
  spline S33 degree 2 poles (7.5878, 156.2375) (7.5878, 155.8408) (7.3337, 155.1634) (7.102, 154.9138) knots 0 0 0 1 2 2 2
  spline S34 degree 2 poles (7.102, 154.9138) (6.8702, 154.6642) (6.1794, 154.3745) (5.7515, 154.3745) knots 0 0 0 1 2 2 2
  spline S35 degree 2 poles (5.7515, 154.3745) (5.3593, 154.3745) (4.5927, 154.5483) (4.3119, 154.6865) knots 0 0 0 1 2 2 2
  line L90 (4.3119, 154.6865) -> (4.3119, 155.4664)
  line L91 (4.3119, 155.4664) -> (4.3653, 155.4664)
  spline S36 degree 2 poles (4.3653, 155.4664) (4.45, 155.404) (4.7665, 155.2436) (4.9581, 155.1723) knots 0 0 0 1 2 2 2
  spline S37 degree 2 poles (4.9581, 155.1723) (5.1765, 155.0965) (5.5375, 155.0118) (5.7649, 155.0118) knots 0 0 0 1 2 2 2
  spline S38 degree 2 poles (5.7649, 155.0118) (5.9877, 155.0118) (6.4067, 155.1723) (6.5582, 155.3461) knots 0 0 0 1 2 2 2
  spline S39 degree 2 poles (6.5582, 155.3461) (6.6964, 155.511) (6.839, 155.9478) (6.839, 156.242) knots 0 0 0 1 2 2 2
  spline S40 degree 2 poles (6.839, 156.242) (6.839, 156.5361) (6.6786, 156.9105) (6.527, 157.0353) knots 0 0 0 1 2 2 2
  spline S41 degree 2 poles (6.527, 157.0353) (6.371, 157.1735) (5.9075, 157.2894) (5.6267, 157.2894) knots 0 0 0 1 2 2 2
  spline S42 degree 2 poles (5.6267, 157.2894) (5.3236, 157.2894) (4.7219, 157.1958) (4.5392, 157.1557) knots 0 0 0 1 2 2 2
  line L92 (4.5392, 157.1557) -> (4.5392, 159.9903)
  line L93 (4.5392, 159.9903) -> (7.5566, 159.9903)
  line L94 (7.5566, 159.9903) -> (7.5566, 159.3441)
  line L95 (7.5566, 159.3441) -> (5.2478, 159.3441)
  line L96 (5.2478, 159.3441) -> (5.2478, 157.8777)
  spline S43 degree 2 poles (5.2478, 157.8777) (5.3816, 157.8955) (5.6401, 157.9089) (5.747, 157.9089) knots 0 0 0 1 2 2 2
  spline S44 degree 2 poles (5.747, 157.9089) (6.1705, 157.9089) (6.7543, 157.7707) (7.0217, 157.5657) knots 0 0 0 1 2 2 2
  spline S45 degree 2 poles (7.0217, 157.5657) (7.2936, 157.3607) (7.5878, 156.7367) (7.5878, 156.2375) knots 0 0 0 1 2 2 2
  spline S46 degree 2 poles (11.8042, 157.2403) (11.8042, 155.7606) (10.944, 154.3745) (10.0481, 154.3745) knots 0 0 0 1 2 2 2
  spline S47 degree 2 poles (10.0481, 154.3745) (9.1388, 154.3745) (8.2875, 155.7874) (8.2875, 157.2359) knots 0 0 0 1 2 2 2
  spline S48 degree 2 poles (8.2875, 157.2359) (8.2875, 158.7245) (9.1478, 160.1018) (10.0481, 160.1018) knots 0 0 0 1 2 2 2
  spline S49 degree 2 poles (10.0481, 160.1018) (10.9529, 160.1018) (11.8042, 158.6755) (11.8042, 157.2403) knots 0 0 0 1 2 2 2
  spline S50 degree 2 poles (10.8593, 155.5645) (10.9662, 155.8364) (11.0554, 156.6743) (11.0554, 157.2403) knots 0 0 0 1 2 2 2
  spline S51 degree 2 poles (11.0554, 157.2403) (11.0554, 157.8064) (10.9662, 158.6399) (10.8548, 158.9207) knots 0 0 0 1 2 2 2
  spline S52 degree 2 poles (10.8548, 158.9207) (10.7434, 159.2015) (10.3556, 159.4912) (10.0481, 159.4912) knots 0 0 0 1 2 2 2
  spline S53 degree 2 poles (10.0481, 159.4912) (9.7405, 159.4912) (9.3439, 159.2015) (9.228, 158.9117) knots 0 0 0 1 2 2 2
  spline S54 degree 2 poles (9.228, 158.9117) (9.1166, 158.6309) (9.0363, 157.7752) (9.0363, 157.2359) knots 0 0 0 1 2 2 2
  spline S55 degree 2 poles (9.0363, 157.2359) (9.0363, 156.6565) (9.1076, 155.8809) (9.2235, 155.5779) knots 0 0 0 1 2 2 2
  spline S56 degree 2 poles (9.2235, 155.5779) (9.3305, 155.2926) (9.7272, 154.9851) (10.0481, 154.9851) knots 0 0 0 1 2 2 2
  spline S57 degree 2 poles (10.0481, 154.9851) (10.3512, 154.9851) (10.7478, 155.2748) (10.8593, 155.5645) knots 0 0 0 1 2 2 2
  line L97 (3.2147, 144.536) -> (0.5316, 144.536)
  line L98 (0.5316, 144.536) -> (0.5316, 145.0976)
  line L99 (0.5316, 145.0976) -> (1.53, 145.0976)
  line L100 (1.53, 145.0976) -> (1.53, 148.7836)
  line L101 (1.53, 148.7836) -> (0.5316, 148.7836)
  line L102 (0.5316, 148.7836) -> (0.5316, 149.2872)
  spline S58 degree 2 poles (0.5316, 149.2872) (1.0976, 149.2872) (1.6325, 149.6081) (1.6681, 150.0538) knots 0 0 0 1 2 2 2
  line L103 (1.6681, 150.0538) -> (2.2386, 150.0538)
  line L104 (2.2386, 150.0538) -> (2.2386, 145.0976)
  line L105 (2.2386, 145.0976) -> (3.2147, 145.0976)
  line L106 (3.2147, 145.0976) -> (3.2147, 144.536)
  spline S59 degree 2 poles (5.7107, 149.5145) (5.5101, 149.5145) (5.1134, 149.4165) (4.9218, 149.3407) knots 0 0 0 1 2 2 2
  spline S60 degree 2 poles (4.9218, 149.3407) (4.7435, 149.2649) (4.4805, 149.1045) (4.378, 149.0332) knots 0 0 0 1 2 2 2
  line L107 (4.378, 149.0332) -> (4.3334, 149.0332)
  line L108 (4.3334, 149.0332) -> (4.3334, 149.8132)
  spline S61 degree 2 poles (4.3334, 149.8132) (4.5741, 149.9424) (5.3987, 150.1519) (5.7686, 150.1519) knots 0 0 0 1 2 2 2
  spline S62 degree 2 poles (5.7686, 150.1519) (6.143, 150.1519) (6.7001, 150.0004) (6.9274, 149.8399) knots 0 0 0 1 2 2 2
  spline S63 degree 2 poles (6.9274, 149.8399) (7.1681, 149.6661) (7.4177, 149.1624) (7.4177, 148.8237) knots 0 0 0 1 2 2 2
  spline S64 degree 2 poles (7.4177, 148.8237) (7.4177, 148.3691) (6.8205, 147.6827) (6.4015, 147.5935) knots 0 0 0 1 2 2 2
  line L109 (6.4015, 147.5935) -> (6.4015, 147.5401)
  spline S65 degree 2 poles (6.4015, 147.5401) (6.5753, 147.5044) (6.972, 147.344) (7.1414, 147.1835) knots 0 0 0 1 2 2 2
  spline S66 degree 2 poles (7.1414, 147.1835) (7.3107, 147.0275) (7.5247, 146.5283) (7.5247, 146.1673) knots 0 0 0 1 2 2 2
  spline S67 degree 2 poles (7.5247, 146.1673) (7.5247, 145.7974) (7.2706, 145.1689) (7.0389, 144.9282) knots 0 0 0 1 2 2 2
  spline S68 degree 2 poles (7.0389, 144.9282) (6.7982, 144.6786) (6.1163, 144.4201) (5.6839, 144.4201) knots 0 0 0 1 2 2 2
  spline S69 degree 2 poles (5.6839, 144.4201) (5.2694, 144.4201) (4.4582, 144.6207) (4.1819, 144.7589) knots 0 0 0 1 2 2 2
  line L110 (4.1819, 144.7589) -> (4.1819, 145.5388)
  line L111 (4.1819, 145.5388) -> (4.2354, 145.5388)
  spline S70 degree 2 poles (4.2354, 145.5388) (4.4671, 145.3695) (5.2516, 145.0575) (5.6394, 145.0575) knots 0 0 0 1 2 2 2
  spline S71 degree 2 poles (5.6394, 145.0575) (5.8667, 145.0575) (6.3213, 145.2001) (6.4728, 145.365) knots 0 0 0 1 2 2 2
  spline S72 degree 2 poles (6.4728, 145.365) (6.6199, 145.5299) (6.7759, 145.9222) (6.7759, 146.2208) knots 0 0 0 1 2 2 2
  spline S73 degree 2 poles (6.7759, 146.2208) (6.7759, 146.5194) (6.6021, 146.9072) (6.4461, 147.0186) knots 0 0 0 1 2 2 2
  spline S74 degree 2 poles (6.4461, 147.0186) (6.2901, 147.13) (5.8667, 147.2147) (5.6171, 147.2147) knots 0 0 0 1 2 2 2
  line L112 (5.6171, 147.2147) -> (5.3051, 147.2147)
  line L113 (5.3051, 147.2147) -> (5.3051, 147.8253)
  line L114 (5.3051, 147.8253) -> (5.5502, 147.8253)
  spline S75 degree 2 poles (5.5502, 147.8253) (6.0449, 147.8253) (6.6689, 148.2978) (6.6689, 148.7479) knots 0 0 0 1 2 2 2
  spline S76 degree 2 poles (6.6689, 148.7479) (6.6689, 148.9574) (6.5085, 149.256) (6.3792, 149.3452) knots 0 0 0 1 2 2 2
  spline S77 degree 2 poles (6.3792, 149.3452) (6.2411, 149.4388) (5.9023, 149.5145) (5.7107, 149.5145) knots 0 0 0 1 2 2 2
  spline S78 degree 2 poles (11.7767, 147.286) (11.7767, 145.8063) (10.9165, 144.4201) (10.0206, 144.4201) knots 0 0 0 1 2 2 2
  spline S79 degree 2 poles (10.0206, 144.4201) (9.1114, 144.4201) (8.2601, 145.833) (8.2601, 147.2816) knots 0 0 0 1 2 2 2
  spline S80 degree 2 poles (8.2601, 147.2816) (8.2601, 148.7702) (9.1203, 150.1474) (10.0206, 150.1474) knots 0 0 0 1 2 2 2
  spline S81 degree 2 poles (10.0206, 150.1474) (10.9254, 150.1474) (11.7767, 148.7212) (11.7767, 147.286) knots 0 0 0 1 2 2 2
  spline S82 degree 2 poles (10.8318, 145.6102) (10.9388, 145.882) (11.0279, 146.72) (11.0279, 147.286) knots 0 0 0 1 2 2 2
  spline S83 degree 2 poles (11.0279, 147.286) (11.0279, 147.8521) (10.9388, 148.6855) (10.8274, 148.9663) knots 0 0 0 1 2 2 2
  spline S84 degree 2 poles (10.8274, 148.9663) (10.7159, 149.2471) (10.3282, 149.5368) (10.0206, 149.5368) knots 0 0 0 1 2 2 2
  spline S85 degree 2 poles (10.0206, 149.5368) (9.7131, 149.5368) (9.3164, 149.2471) (9.2005, 148.9574) knots 0 0 0 1 2 2 2
  spline S86 degree 2 poles (9.2005, 148.9574) (9.0891, 148.6766) (9.0089, 147.8209) (9.0089, 147.2816) knots 0 0 0 1 2 2 2
  spline S87 degree 2 poles (9.0089, 147.2816) (9.0089, 146.7021) (9.0802, 145.9266) (9.1961, 145.6235) knots 0 0 0 1 2 2 2
  spline S88 degree 2 poles (9.1961, 145.6235) (9.303, 145.3383) (9.6997, 145.0307) (10.0206, 145.0307) knots 0 0 0 1 2 2 2